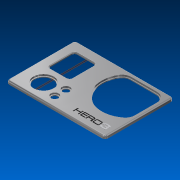
# Autodesk Inventor part: GoPro Hero 3 Front Panel
Saved by Autodesk Inventor 2015 (Build 190159000, 159)
## iProperties
Created: 2013-02-14
Material: ABS Plastic
Document SubType Name: Modeling
Designer: sdarley
Density: 1 g/cm^3
Project: GoPro Hero 3 HD Camera
Description: GoPro Hero 3 Front Panel
Appearance: Silver
Author: sdarley
Title: GoPro Hero 3 Front Panel
Revision Number: 1
Autodesk Inventor part; units mm, degrees
ref_plane "YZ Plane" through (0, 0, 0) normal (1, 0, 0) x (0, 1, 0)
ref_plane "XZ Plane" through (0, 0, 0) normal (0, 1, 0) x (-1, 0, 0)
ref_plane "XY Plane" through (0, 0, 0) normal (0, 0, 1) x (1, 0, 0)
sketch "Sketch1" plane through (0, 0, 0) normal (0, 0, 1) x (1, 0, 0)
  line L0 (-29.625, -20.6) -> (29.625, -20.6)
  line L1 (29.625, -20.6) -> (29.625, 20.6)
  line L2 (29.625, 20.6) -> (-29.625, 20.6)
  line L3 (-29.625, 20.6) -> (-29.625, -20.6)
  line L4 (-29.625, -20.6) -> (29.625, 20.6) construction
  line L5 (29.625, -20.6) -> (-29.625, 20.6) construction
  line L6 (-23.825, 14.6) -> (-10.825, 14.6)
  line L7 (-10.825, 14.6) -> (-10.825, -1.4)
  line L8 (-10.825, -1.4) -> (-23.825, -1.4)
  line L9 (-23.825, -1.4) -> (-23.825, 14.6)
  circle A0 centre (-17.025, -10.8) radius 6.075
  circle A1 centre (-6.725, -7.65) radius 2.4
  circle A2 centre (-6.725, -14.4) radius 2.4
  line L10 (6.353, 18.3) -> (21.925, 18.3)
  line L11 (27.425, 12.8) -> (27.425, -0.6854)
  arc A3 (1.5749, 15.5238) -> (25.3036, -5.0253) centre (15.475, 7.6) ccw
  arc A4 (6.353, 18.3) -> (1.5749, 15.5238) centre (6.353, 12.8) ccw
  arc A5 (25.3036, -5.0253) -> (27.425, -0.6854) centre (21.925, -0.6854) ccw
  arc A6 (27.425, 12.8) -> (21.925, 18.3) centre (21.925, 12.8) ccw
  point P0 (0, 0)
  point P1 (3.5792, 18.3)
  point P2 (27.425, -3.0394)
  dimension "d0" = 59.25
  dimension "d1" = 41.2
  dimension "d6" = 13
  dimension "d7" = 16
  dimension "d8" = 6
  dimension "d9" = 5.8
  dimension "d12" = 4.8
  dimension "d13" = 6.2
  dimension "d14" = 6.75
  dimension "d15" = 22.9
  dimension "d16" = 12.15
  dimension "d17" = 12.6
  dimension "d18" = 9.8
  dimension "d19" = 5.5
  dimension "d20" = 5.5
  dimension "d21" = 2.2
  dimension "d22" = 2.3
  dimension "d23" = 30.15
  dimension "d24" = 29
  dimension "d25" = 16
  constraints: 24 end point, 10 point on circle, 7 centre point, 6 tangent, 4 parallel, 4 perpendicular, 2 equal radius, 2 horizontal, 2 midpoint, 2 point on line, 1 vertical alignment
  measures "d0" distance of L2.end L1.end
  measures "d1" distance of L1.end L0.end
  measures "d6" distance of L7.end L8.end
  measures "d7" distance of L6.end L7.end
  measures "d8" distance between parallel lines of L2 L6
  measures "d9" distance between parallel lines of L3 L9
  measures "d12" diameter of A1
  measures "d13" distance from line of A2.centre L0
  measures "d14" distance of A1.centre A2.centre
  measures "d15" distance from line of L3 A2.centre
  measures "d16" diameter of A0
  measures "d17" distance from line of A0.centre L3
  measures "d18" distance from line of A0.centre L0
  measures "d19" radius of A4
  measures "d20" radius of A6
  measures "d21" distance between parallel lines of L1 L11
  measures "d22" distance between parallel lines of L10 L2
  measures "d25" radius of A3
extrude "Extrusion1" add sketch "Sketch1" along normal blind 1.75
fillet "Fillet1" radius 1.75 4 edges at (29.625, 20.6, 0.875) (-29.625, 20.6, 0.875) (-29.625, -20.6, 0.875) (29.625, -20.6, 0.875)
fillet "Fillet2" radius 0.95 8 edges at (29.1124, 20.0874, 1.75) (0, 20.6, 1.75) (-29.1124, 20.0874, 1.75) (-29.625, 0, 1.75) (-29.1124, -20.0874, 1.75) (0, -20.6, 1.75) (29.1124, -20.0874, 1.75) (29.625, 0, 1.75)
fillet "Fillet3" radius 1.6 4 edges at (-23.825, 14.6, 0.875) (-10.825, 14.6, 0.875) (-23.825, -1.4, 0.875) (-10.825, -1.4, 0.875)
fillet "Fillet4" radius 0.5 8 edges at (-23.3564, 14.1314, 1.75) (-17.325, 14.6, 1.75) (-11.2936, 14.1314, 1.75) (-10.825, 6.6, 1.75) (-11.2936, -0.9314, 1.75) (-17.325, -1.4, 1.75) (-23.3564, -0.9314, 1.75) (-23.825, 6.6, 1.75)
sketch "Sketch2" plane through (0, 0, 0) normal (0, 0, -1) x (-1, 0, 0)
  line L0 (-21.925, 18.3) -> (-6.353, 18.3) projected
  arc A0 (-1.5749, 15.5238) -> (-6.353, 18.3) centre (-6.353, 12.8) ccw projected
  arc A1 (-25.3036, -5.0253) -> (-1.5749, 15.5238) centre (-15.475, 7.6) ccw projected
  arc A2 (-27.425, -0.6854) -> (-25.3036, -5.0253) centre (-21.925, -0.6854) ccw projected
  line L1 (-27.425, -0.6854) -> (-27.425, 12.8) projected
  arc A3 (-21.925, 18.3) -> (-27.425, 12.8) centre (-21.925, 12.8) ccw projected
  line L2 (10.825, 0.2) -> (10.825, 13) projected
  arc A4 (12.425, 14.6) -> (10.825, 13) centre (12.425, 13) ccw projected
  line L3 (12.425, 14.6) -> (22.225, 14.6) projected
  arc A5 (23.825, 13) -> (22.225, 14.6) centre (22.225, 13) ccw projected
  line L4 (23.825, 13) -> (23.825, 0.2) projected
  arc A6 (22.225, -1.4) -> (23.825, 0.2) centre (22.225, 0.2) ccw projected
  line L5 (22.225, -1.4) -> (12.425, -1.4) projected
  arc A7 (10.825, 0.2) -> (12.425, -1.4) centre (12.425, 0.2) ccw projected
  circle A8 centre (17.025, -10.8) radius 6.075 projected
  circle A9 centre (6.725, -14.4) radius 2.4 projected
  circle A10 centre (6.725, -7.65) radius 2.4 projected
  arc A11 (-29.625, -18.85) -> (-27.875, -20.6) centre (-27.875, -18.85) ccw projected
  line L6 (27.875, -20.6) -> (-27.875, -20.6) projected
  arc A12 (27.875, -20.6) -> (29.625, -18.85) centre (27.875, -18.85) ccw projected
  line L7 (29.625, 18.85) -> (29.625, -18.85) projected
  arc A13 (29.625, 18.85) -> (27.875, 20.6) centre (27.875, 18.85) ccw projected
  line L8 (-27.875, 20.6) -> (27.875, 20.6) projected
  arc A14 (-27.875, 20.6) -> (-29.625, 18.85) centre (-27.875, 18.85) ccw projected
  line L9 (-29.625, -18.85) -> (-29.625, 18.85) projected
  arc A15 (28.875, 18.85) -> (27.875, 19.85) centre (27.875, 18.85) ccw
  line L10 (28.875, 18.85) -> (28.875, -18.85)
  arc A16 (27.875, -19.85) -> (28.875, -18.85) centre (27.875, -18.85) ccw
  line L11 (27.875, -19.85) -> (-27.875, -19.85)
  arc A17 (-28.875, -18.85) -> (-27.875, -19.85) centre (-27.875, -18.85) ccw
  line L12 (-28.875, -18.85) -> (-28.875, 18.85)
  arc A18 (-27.875, 19.85) -> (-28.875, 18.85) centre (-27.875, 18.85) ccw
  line L13 (-27.875, 19.85) -> (27.875, 19.85)
  point P0 (0, 0)
  dimension "d26" = 0.75
  constraints: 8 end point, 8 point on circle, 4 centre point, 7 other
  measures "d26" distance between parallel lines of L8 L13
extrude "Extrusion2" cut sketch "Sketch2" against normal blind 0.8 contours L10 A16 L11 A17 L12 A18 L13 A15
sketch "Sketch3" plane through (0, 0, 0.8) normal (0, 0, -1) x (-1, 0, 0)
  arc A0 (-21.925, 18.3) -> (-27.425, 12.8) centre (-21.925, 12.8) ccw projected
  line L0 (-6.353, 18.3) -> (-21.925, 18.3) projected
  arc A1 (-1.5749, 15.5238) -> (-6.353, 18.3) centre (-6.353, 12.8) ccw projected
  arc A2 (-25.3036, -5.0253) -> (-1.5749, 15.5238) centre (-15.475, 7.6) ccw projected
  arc A3 (-27.425, -0.6854) -> (-25.3036, -5.0253) centre (-21.925, -0.6854) ccw projected
  line L1 (-27.425, 12.8) -> (-27.425, -0.6854) projected
  circle A4 centre (17.025, -10.8) radius 6.075 projected
  circle A5 centre (6.725, -7.65) radius 2.4 projected
  circle A6 centre (6.725, -14.4) radius 2.4 projected
  line L2 (-6.353, 17.8) -> (-21.925, 17.8)
  arc A7 (-21.925, 17.8) -> (-26.925, 12.8) centre (-21.925, 12.8) ccw
  line L3 (-26.925, 12.8) -> (-26.925, -0.6854)
  arc A8 (-26.925, -0.6854) -> (-24.9964, -4.6308) centre (-21.925, -0.6854) ccw
  arc A9 (-24.9964, -4.6308) -> (-2.0093, 15.2762) centre (-15.475, 7.6) ccw
  arc A10 (-2.0093, 15.2762) -> (-6.353, 17.8) centre (-6.353, 12.8) ccw
  circle A11 centre (6.725, -7.65) radius 1.9
  circle A12 centre (6.725, -14.4) radius 1.9
  circle A13 centre (17.025, -10.8) radius 5.575
  point P0 (0, 0)
  dimension "d29" = 0.5
  dimension "d30" = 0.5
  dimension "d31" = 0.5
  dimension "d32" = 0.5
  constraints: 8 point on circle, 7 centre point, 4 end point, 5 other
  measures "d29" radial gap between concentric circles of A11 A5
  measures "d30" radial gap between concentric circles of A12 A6
  measures "d31" radial gap between concentric circles of A4 A13
  measures "d32" radial gap between concentric circles of A2 A9
extrude "Extrusion3" add sketch "Sketch3" along normal blind 0.5
sketch "Sketch4" plane through (0, 0, 1.75) normal (0, 0, 1) x (1, 0, 0)
  line L0 (-27.875, 19.65) -> (27.875, 19.65) projected
  line L1 (27.875, 20.6) -> (-27.875, 20.6) projected
  arc A0 (-27.875, 20.6) -> (-29.625, 18.85) centre (-27.875, 18.85) ccw projected
  line L2 (-29.625, 18.85) -> (-29.625, -18.85) projected
  arc A1 (-29.625, -18.85) -> (-27.875, -20.6) centre (-27.875, -18.85) ccw projected
  line L3 (-27.875, -20.6) -> (27.875, -20.6) projected
  arc A2 (27.875, -20.6) -> (29.625, -18.85) centre (27.875, -18.85) ccw projected
  line L4 (29.625, -18.85) -> (29.625, 18.85) projected
  arc A3 (29.625, 18.85) -> (27.875, 20.6) centre (27.875, 18.85) ccw projected
  line L5 (13.6484, -13.8195) -> (13.6484, -14.302)
  line L6 (13.6484, -14.302) -> (11.2852, -14.302)
  line L7 (11.2852, -14.302) -> (11.2852, -14.9825)
  line L8 (11.2852, -14.9825) -> (13.6484, -14.9825)
  line L9 (13.6484, -14.9825) -> (13.6484, -15.5146)
  line L10 (13.6484, -15.5146) -> (11.2852, -15.5146)
  line L11 (11.2852, -15.5146) -> (11.2852, -16.3435)
  line L12 (11.2852, -16.3435) -> (13.6484, -16.3435)
  line L13 (13.6484, -16.3435) -> (13.6484, -16.875)
  line L14 (13.6484, -16.875) -> (10.7903, -16.875)
  line L15 (10.7903, -16.875) -> (10.7903, -13.8195)
  line L16 (10.7903, -13.8195) -> (13.6484, -13.8195)
  line L17 (14.0868, -13.7999) -> (14.0868, -16.875)
  line L18 (14.0868, -16.875) -> (14.5658, -16.875)
  line L19 (14.5658, -16.875) -> (14.5658, -15.663)
  line L20 (14.5658, -15.663) -> (16.6403, -15.663)
  line L21 (10.0858, -13.8195) -> (10.0858, -16.875)
  line L22 (10.0858, -16.875) -> (9.6033, -16.875)
  line L23 (9.6033, -16.875) -> (9.6033, -15.4898)
  line L24 (9.6033, -15.4898) -> (7.0414, -15.4898)
  line L25 (7.0414, -15.4898) -> (7.0414, -16.875)
  line L26 (7.0414, -16.875) -> (6.5713, -16.875)
  line L27 (6.5713, -16.875) -> (6.5713, -13.8195)
  line L28 (6.5713, -13.8195) -> (7.0414, -13.8195)
  line L29 (7.0414, -13.8195) -> (7.0414, -14.9825)
  line L30 (7.0414, -14.9825) -> (9.6026, -14.9825)
  line L31 (9.6026, -14.9825) -> (9.6026, -13.8195)
  line L32 (9.6026, -13.8195) -> (10.0858, -13.8195)
  line L33 (14.0868, -13.7999) -> (16.7221, -13.7999)
  line L34 (16.9109, -15.981) -> (16.9109, -16.875)
  line L35 (16.9109, -16.875) -> (17.6069, -16.875)
  line L36 (17.6069, -16.875) -> (17.6069, -15.9871)
  line L37 (14.5658, -14.302) -> (14.5658, -15.1488)
  line L38 (14.5658, -15.1488) -> (16.5064, -15.1488)
  line L39 (14.5658, -14.302) -> (16.5064, -14.302)
  arc A4 (16.5064, -15.1488) -> (16.5064, -14.302) centre (16.5064, -14.7254) ccw
  arc A5 (17.1174, -15.4563) -> (16.7221, -13.7999) centre (16.7221, -14.6753) ccw
  arc A6 (17.6069, -15.9871) -> (17.1174, -15.4563) centre (17.0744, -15.9871) ccw
  arc A7 (16.9109, -15.981) -> (16.6403, -15.663) centre (16.6403, -15.9371) ccw
  line L40 (18.7394, -13.7999) -> (21.1202, -13.7999)
  line L41 (18.804, -14.302) -> (21.0955, -14.302)
  line L42 (18.804, -16.3435) -> (21.0955, -16.3435)
  line L43 (21.1202, -16.875) -> (18.7394, -16.875)
  line L44 (18.0741, -14.4652) -> (18.0741, -16.2097)
  line L45 (18.521, -14.585) -> (18.521, -16.0606)
  line L46 (21.3785, -14.585) -> (21.3785, -16.0606)
  line L47 (21.7855, -14.4652) -> (21.7855, -16.2097)
  arc A8 (18.804, -14.302) -> (18.521, -14.585) centre (18.804, -14.585) ccw
  arc A9 (21.3785, -14.585) -> (21.0955, -14.302) centre (21.0955, -14.585) ccw
  arc A10 (21.7855, -14.4652) -> (21.1202, -13.7999) centre (21.1202, -14.4652) ccw
  arc A11 (18.7394, -13.7999) -> (18.0741, -14.4652) centre (18.7394, -14.4652) ccw
  arc A12 (18.0741, -16.2097) -> (18.7394, -16.875) centre (18.7394, -16.2097) ccw
  arc A13 (21.1202, -16.875) -> (21.7855, -16.2097) centre (21.1202, -16.2097) ccw
  arc A14 (21.0955, -16.3435) -> (21.3785, -16.0606) centre (21.0955, -16.0606) ccw
  arc A15 (18.521, -16.0606) -> (18.804, -16.3435) centre (18.804, -16.0606) ccw
  line L48 (22.2148, -14.7133) -> (23.179, -14.7133)
  line L49 (23.5754, -13.3526) -> (25.4114, -13.3526)
  line L50 (23.7403, -14.152) -> (25.1357, -14.152)
  line L51 (22.2148, -15.6024) -> (23.179, -15.6024)
  line L52 (23.5754, -16.9631) -> (25.4114, -16.9631)
  line L53 (23.7403, -16.1636) -> (25.1357, -16.1636)
  arc A16 (23.5754, -13.3526) -> (22.2148, -14.7133) centre (23.5754, -14.7133) ccw
  arc A17 (23.7403, -14.152) -> (23.179, -14.7133) centre (23.7403, -14.7133) ccw
  arc A18 (25.6703, -15.1578) -> (25.4114, -13.3526) centre (25.4114, -14.2738) ccw
  arc A19 (25.4114, -16.9631) -> (25.6703, -15.1578) centre (25.4114, -16.0419) ccw
  arc A20 (25.1357, -16.1636) -> (25.1357, -15.4176) centre (25.1357, -15.7906) ccw
  arc A21 (25.1357, -14.8981) -> (25.1357, -14.152) centre (25.1357, -14.5251) ccw
  arc A22 (23.179, -15.6024) -> (23.7403, -16.1636) centre (23.7403, -15.6024) ccw
  arc A23 (22.2148, -15.6024) -> (23.5754, -16.9631) centre (23.5754, -15.6024) ccw
  line L54 (23.9377, -14.8981) -> (23.9377, -15.4176)
  line L55 (23.9377, -15.4176) -> (25.1357, -15.4176)
  line L56 (23.9377, -14.8981) -> (25.1357, -14.8981)
  point P0 (0, 0)
  point P1 (23.9377, -15.1578)
  constraints: 104 end point, 42 point on circle, 37 parallel, 31 tangent, 20 centre point, 19 horizontal, 19 vertical, 12 perpendicular, 10 equal radius, 8 horizontal alignment, 4 line through centre, 3 collinear, 2 vertical alignment, 1 midpoint, 13 other
emboss "Emboss1" sketch "Sketch4" operation add depth 0.1 direction (0, 0, -1) contours L5 L6 L7 L8 L9 L10 L11 L12 L13 L14 L15 L16 | L33 A5 A6 L36 L35 L34 A7 L20 L19 L18 L17 | L21 L22 L23 L24 L25 L26 L27 L28 L29 L30 L31 L32 | L40 A10 L47 A13 L43 A12 L44 A11
sketch "Sketch5" plane through (0, 0, 1.75) normal (0, 0, 1) x (1, 0, 0)
  line L0 (21.1202, -16.875) -> (18.7394, -16.875) projected
  arc A0 (23.5478, -13.3489) -> (22.1981, -14.6986) centre (23.5478, -14.6986) ccw
  arc A1 (23.7088, -14.1616) -> (23.1719, -14.6986) centre (23.7088, -14.6986) ccw
  line L1 (22.1981, -14.6986) -> (23.1719, -14.6986)
  line L2 (23.7088, -14.1616) -> (25.1316, -14.1616)
  line L3 (23.5478, -13.3489) -> (25.3931, -13.3489)
  line L4 (23.9333, -14.9014) -> (25.1316, -14.9014)
  line L5 (23.9333, -14.9014) -> (23.9333, -15.4172)
  line L6 (23.9333, -15.4172) -> (25.1316, -15.4172)
  arc A2 (25.1316, -14.9014) -> (25.1316, -14.1616) centre (25.1316, -14.5315) ccw
  line L7 (22.1981, -15.5961) -> (23.1719, -15.5961)
  line L8 (23.7083, -16.157) -> (25.1316, -16.157)
  arc A3 (25.1316, -16.157) -> (25.1316, -15.4172) centre (25.1316, -15.7871) ccw
  arc A4 (23.1719, -15.5961) -> (23.7083, -16.157) centre (23.7083, -15.62) ccw
  line L9 (23.5817, -16.9796) -> (25.3931, -16.9796)
  arc A5 (25.6685, -15.1593) -> (25.3931, -13.3489) centre (25.3931, -14.275) ccw
  arc A6 (25.3931, -16.9796) -> (25.6685, -15.1593) centre (25.3931, -16.0486) ccw
  arc A7 (22.1981, -15.5961) -> (23.5817, -16.9796) centre (23.5817, -15.5961) ccw
  point P0 (0, 0)
  point P1 (23.9333, -15.1593)
  constraints: 18 end point, 17 point on circle, 10 tangent, 8 centre point, 8 horizontal, 7 parallel, 4 vertical alignment, 3 line through centre, 2 equal radius, 2 perpendicular, 1 horizontal alignment, 1 midpoint, 1 vertical, 34 other
emboss "Emboss2" sketch "Sketch5" operation add depth 0.1 direction (0, 0, -1)
ref_plane "Work Plane1" through (-17.025, -18.85, 0) normal (-1, 0, 0) x (0, 0, 1)
equation "\"d30\" = d29"
equation "\"d31\" = d29"
equation "\"d32\" = d29"
body "Solid1"
